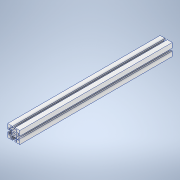
# Autodesk Inventor part: Horizontal
Saved by Autodesk Inventor 2021 (Build 250183000, 183)
## iProperties
Created: 2020-10-09
Part Number: Horizontal
Material: Aluminio 6061
Document SubType Name: Modeling
Designer: juanm
Density: 2.7 g/cm^3
Appearance: Aluminio - Plano
Author: juanm
Autodesk Inventor part; units mm, degrees
ref_plane "YZ Plane" through (0, 0, 0) normal (1, 0, 0) x (0, 1, 0)
ref_plane "XZ Plane" through (0, 0, 0) normal (0, 1, 0) x (-1, 0, 0)
ref_plane "XY Plane" through (0, 0, 0) normal (0, 0, 1) x (1, 0, 0)
sketch "Boceto2" plane through (0, 0, 0) normal (0, 0, 1) x (1, 0, 0)
  line L0 (29.6723, -57.4121) -> (29.6723, -41.4123)
  line L1 (29.6723, -41.4123) -> (34.1724, -41.4123)
  line L2 (34.1534, -41.4123) -> (34.1534, -44.4122)
  arc A0 (34.1534, -44.4122) -> (34.1534, -47.4122) centre (34.1534, -45.9122) ccw
  line L3 (34.1534, -47.4122) -> (38.1534, -47.4122)
  line L4 (38.1534, -47.4122) -> (41.9534, -43.6122)
  line L5 (29.6724, -33.4123) -> (34.1724, -33.4122)
  line L6 (34.1534, -33.4122) -> (34.1534, -30.4123)
  arc A1 (34.1534, -27.4123) -> (34.1534, -30.4123) centre (34.1534, -28.9123) ccw
  line L7 (34.1534, -27.4123) -> (38.1534, -27.4122)
  line L8 (38.1534, -27.4122) -> (41.9534, -31.2122)
  line L9 (41.9534, -43.6122) -> (41.9534, -31.2122)
  circle A2 centre (49.6724, -37.4122) radius 4.5495
  line L10 (43.4724, -29.6933) -> (55.8724, -29.6933)
  line L11 (45.6723, -21.8933) -> (42.6724, -21.8933)
  line L12 (39.6724, -21.8933) -> (39.6724, -25.8933)
  line L13 (39.6724, -25.8933) -> (43.4724, -29.6933)
  arc A3 (42.6724, -21.8933) -> (39.6724, -21.8933) centre (41.1724, -21.8933) ccw
  line L14 (53.6723, -21.8933) -> (56.6723, -21.8932)
  line L15 (59.6723, -21.8932) -> (59.6723, -25.8932)
  arc A4 (59.6723, -21.8932) -> (56.6723, -21.8932) centre (58.1723, -21.8932) ccw
  line L16 (59.6723, -25.8932) -> (55.8724, -29.6933)
  line L17 (45.6723, -17.4121) -> (45.6723, -21.9122)
  line L18 (53.6723, -17.4123) -> (53.6723, -21.9122)
  circle A5 centre (49.6724, -37.4122) radius 4.5495
  line L19 (57.3913, -31.2122) -> (57.3913, -43.6122)
  line L20 (65.1913, -33.4121) -> (65.1913, -30.4122)
  line L21 (65.1913, -27.4122) -> (61.1913, -27.4122)
  line L22 (61.1913, -27.4122) -> (57.3913, -31.2122)
  arc A6 (65.1913, -30.4122) -> (65.1913, -27.4122) centre (65.1913, -28.9122) ccw
  line L23 (65.1913, -41.4122) -> (65.1913, -44.4121)
  line L24 (65.1913, -47.4121) -> (61.1913, -47.4122)
  arc A7 (65.1913, -47.4121) -> (65.1913, -44.4121) centre (65.1913, -45.9121) ccw
  line L25 (61.1913, -47.4122) -> (57.3913, -43.6122)
  line L26 (69.6724, -33.4121) -> (65.1723, -33.4121)
  line L27 (69.6723, -41.4121) -> (65.1724, -41.4122)
  circle A8 centre (49.6724, -37.4122) radius 4.5495
  line L28 (55.8724, -45.1311) -> (43.4724, -45.1311)
  line L29 (53.6724, -52.9311) -> (56.6724, -52.9311)
  line L30 (59.6724, -52.9311) -> (59.6724, -48.9311)
  line L31 (59.6724, -48.9311) -> (55.8724, -45.1311)
  arc A9 (56.6724, -52.9311) -> (59.6724, -52.9311) centre (58.1724, -52.9311) ccw
  line L32 (45.6724, -52.9311) -> (42.6724, -52.9312)
  line L33 (39.6724, -52.9312) -> (39.6724, -48.9312)
  arc A10 (39.6724, -52.9312) -> (42.6724, -52.9312) centre (41.1724, -52.9312) ccw
  line L34 (39.6724, -48.9312) -> (43.4724, -45.1311)
  line L35 (53.6724, -57.4123) -> (53.6724, -52.9122)
  line L36 (45.6724, -57.4121) -> (45.6724, -52.9122)
  circle A11 centre (49.6724, -37.4122) radius 4.5495
  line L37 (29.6724, -17.4121) -> (45.6723, -17.4121)
  line L38 (53.6723, -17.4123) -> (69.6724, -17.4123)
  line L39 (29.6724, -33.4123) -> (29.6724, -17.4121)
  line L40 (29.6723, -57.4121) -> (45.6724, -57.4121)
  line L41 (69.6723, -41.4121) -> (69.6723, -57.4123)
  line L42 (69.6723, -57.4123) -> (53.6724, -57.4123)
  line L43 (69.6724, -33.4121) -> (69.6724, -17.4123)
  point P0 (0, 0)
  dimension "d29" = 360
  constraints: 88 end point, 16 point on circle, 12 centre point, 8 point on line, 3 horizontal, 3 perpendicular, 3 vertical, 2 coincident, 1 parallel, 1 tangent, 119 other
extrude "Extrusión2" add sketch "Boceto2" along normal blind 500
